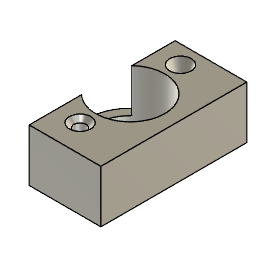
obudowa (Autodesk Fusion 360 archive; units mm, degrees)
design "trzyma_silnik"
Autodesk Fusion 360 part; units mm, degrees
sketch "Sketch1" plane through (0, 0, 0) normal (0, 0, 1) x (1, 0, 0)
  line L0 (22.8277, 15) -> (38.55, 15)
  line L1 (38.55, 15) -> (38.55, -17)
  line L2 (22.8277, -17) -> (22.8277, 15)
  line L3 (38.55, -17) -> (22.8277, -17)
  circle A0 centre (28, 11) radius 1.35
  circle A1 centre (28, 0) radius 7.55
  arc A2 (22.8277, 8.0281) -> (22.8277, -8.0281) centre (28, 0) ccw
  circle A3 centre (28, -11) radius 1.35
  line L4 (22.8277, -39) -> (22.8277, -7)
  point P0 (22.8277, -5.5)
  point P1 (28, 0)
  point P2 (22.8277, 5.5)
  dimension "d27" = 15.1
  dimension "d29" = 10.55
  dimension "d30" = 17
  dimension "d31" = 2.7
  dimension "d32" = 10.55
  dimension "d33" = 15
  dimension "d36" = 11
  dimension "d42" = 0
  dimension "d43" = -22
  constraint coincident P1 A1.centre
  constraint horizontal L0
  constraint vertical L1
  constraint horizontal L3
  constraint vertical L2
  constraint coincident P2 A1
  constraint coincident P2 L2
  constraint coincident P0 A1
  constraint coincident P0 L2
  constraint concentric A1 A2
  constraint coincident L2 A2.end
  constraint coincident L2 A2.start
  measures "d27" diameter of A1
  measures "d29" distance of P1 L1
  measures "d30" distance of P1 L3
  measures "d31" diameter of A0
  measures "d32" distance of A0.centre L1
  measures "d33" distance of P1 L0
  measures "d36" distance of P0 P2
extrude "Extrude1" add sketch "Sketch1" along normal blind 11.5 contours L0 L1 L2 L3 A1 L4
chamfer "Chamfer1" [no effect]
chamfer "Chamfer2" distance 1 distance2 3 1 edges at (26.7414, 11.4882, 11.5) measured on face at (29.8927, -15.4387, 11.5)
chamfer "Chamfer2" distance 1 distance2 1 1 edges at (26.7414, -10.5118, 11.5) measured on face at (29.8927, -15.4387, 11.5)
extrude "Extrude2" add sketch "Sketch1" along normal blind 2 contours L2 A1 A2 L4
equation "d29 = ( 15.1 / 2 ) * 1 mm + 3 mm"

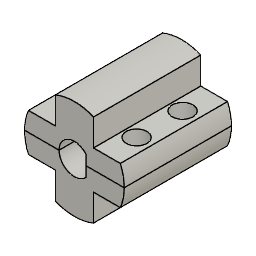
design "laczenie_DC-pret"
part number: laczenie_DC-pret
Autodesk Fusion 360 part; units mm, degrees
sketch "Sketch5" plane through (0, 0, 0) normal (0, 1, 0) x (1, 0, 0)
  circle A0 centre (20, 0) radius 6.5
  circle A1 centre (20, 0) radius 1.45
  line L0 (0, 0) -> (20, 0) construction
  line L1 (20.8832, -1.15) -> (20.8832, 1.15)
  circle A2 centre (20, 0) radius 2
  line L2 (21.5199, -1.3) -> (21.5199, 1.3)
  dimension "d32" = 13
  dimension "d33" = 2.9
  dimension "d34" = 20
  dimension "d37" = 4
  dimension "d39" = 2.6
  dimension "d42" = 2.3
  constraint concentric A0 A1
  constraint coincident L0.start origin
  constraint coincident A0.centre A1.centre
  constraint horizontal L0
  constraint coincident A1 L1.start
  constraint coincident A1 L1.end
  constraint vertical L1
  constraint concentric A1 A2
  constraint coincident A2 L2.start
  constraint coincident A2 L2.end
  constraint parallel L1 L2
  measures "d32" diameter of A0
  measures "d33" diameter of A1
  measures "d34" distance of L0.start A0.centre
  measures "d37" diameter of A2
  measures "d39" distance of L2.start L2.end
  measures "d42" distance of L1.start L1.end
extrude "Extrude9" add sketch "Sketch5" along normal blind 14 contours A0 | A1 L1 | A2 L2 | A2 L2 picked at (21.2814, 0.0105) makes body 1
extrude "Extrude10" cut sketch "Sketch5" along normal blind 7 contours A1 L1 | A2 L2 picked at (21.2814, 0.0105) picked at (18.187, 0) bodies 1
sketch "Sketch6" plane through (0, 0, 0) normal (0, -1, 0) x (1, 0, 0)
  arc A0 (21.5199, 1.3) -> (21.5199, -1.3) centre (20, 0) ccw
  line L0 (21.5199, 1.3) -> (21.5199, -1.3)
  circle A1 centre (20, 0) radius 6.5
  circle A2 centre (20, 0) radius 6.5
  line L1 (17.5, 6) -> (17.5, 2.5)
  line L2 (17.5, 2.5) -> (14, 2.5)
  line L3 (22.5, 6) -> (22.5, 2.5)
  line L4 (22.5, 2.5) -> (26, 2.5)
  line L5 (22.5, -6) -> (22.5, -2.5)
  line L6 (22.5, -2.5) -> (26, -2.5)
  line L7 (17.5, -6) -> (17.5, -2.5)
  line L8 (17.5, -2.5) -> (14, -2.5)
  line L9 (14, 2.5) -> (26, 2.5) construction
  line L10 (14, -2.5) -> (26, -2.5) construction
  line L11 (17.5, 6) -> (17.5, -6) construction
  line L12 (22.5, -6) -> (22.5, 6) construction
  dimension "d45" = 13
  dimension "d46" = 3.5
  constraint concentric A0 A2
  constraint coincident A2 L1.start
  constraint vertical L1
  constraint coincident A1 L2.end
  constraint perpendicular L1 L2
  constraint coincident A2 L3.start
  constraint perpendicular L2 L3
  constraint coincident A1 L4.end
  constraint perpendicular L3 L4
  constraint coincident A2 L5.start
  constraint vertical L5
  constraint coincident A2 L6.end
  constraint perpendicular L5 L6
  constraint coincident A2 L7.start
  constraint perpendicular L6 L7
  constraint coincident A1 L8.end
  constraint perpendicular L7 L8
  constraint perpendicular L3 L9
  constraint parallel L6 L10
  constraint perpendicular L9 L12
  constraint collinear L3 L12
  constraint vertical L11
  constraint equal L9 L12
  constraint equal L9 L11
  constraint equal L10 L11
  measures "d45" diameter of A2
  measures "d46" distance of L1.end L2.end
extrude "Extrude11" cut sketch "Sketch6" against normal blind 22 contours A1 A2 L3 L4 | A1 A2 L5 L6 | A1 A2 L1 L2 | A1 A2 L7 L8 bodies 1
sketch "Sketch7" plane through (0, 0, 2.5) normal (0, 0, 1) x (-1, 0, 0)
  line L0 (-17.5, -14) -> (-14, -14)
  line L1 (-14, -14) -> (-14, 0)
  line L2 (-14, 0) -> (-17.5, 0)
  line L3 (-17.5, 0) -> (-17.5, -14)
  circle A0 centre (-15.925, -10) radius 1.35
  circle A1 centre (-24.12, -10) radius 1.35
  line L4 (-24.12, -10) -> (-24.12, -14) construction
  line L5 (-24.12, -10) -> (-25.82, -10) construction
  line L6 (-15.925, -10) -> (-14.225, -10) construction
  line L7 (-15.925, -10) -> (-15.925, -14) construction
  line L8 (-14, -7) -> (-26, -7) construction
  line L9 (-14, -7) -> (-26, -7) construction
  circle A2 centre (-15.925, -4) radius 1.35
  circle A3 centre (-24.12, -4) radius 1.35
  dimension "d49" = 2.7
  dimension "d50" = 2.7
  dimension "d52" = 4
  dimension "d53" = 1.7
  constraint coincident A1.centre L4.start
  constraint vertical L4
  constraint perpendicular L4 L5
  constraint coincident A0.centre L6.start
  constraint perpendicular L1 L6
  constraint coincident L0 L7.end
  constraint perpendicular L0 L7
  constraint equal L4 L7
  constraint equal L5 L6
  constraint collinear L5 L6
  constraint midpoint L1 L8.start
  constraint perpendicular L1 L8
  constraint symmetric A0 L8 A2
  constraint symmetric A1 L8 A3
  constraint symmetric L9.start L8 L8.start
  constraint symmetric L9.end L8 L8.end
  measures "d49" diameter of A0
  measures "d50" diameter of A1
  measures "d52" distance of A0.centre L7.end
  measures "d53" distance of A0.centre L6.end
extrude "Extrude12" cut sketch "Sketch7" against normal blind 7 contours A0 | A1 | A2 | A3 bodies 1
copy_body "Body->Comp1" bodies 1 removing the originals makes body 2 in component "MaterialInv_072"
ref_plane "WorkPlane1" through (24.25, 7, 0) normal (0, 0, 1) x (1, 0, 0) in component "MaterialInv_072"
split "Split1" by plane through (24.25, 7, 0) normal (0, 0, 1) bodies 2 makes body 3 at (21.4142, 9.3333, 6.3443) in component "MaterialInv_072"
component "MaterialInv_072" placed x (1, 0, 0) y (0, 1, 0) z (0, 0, 1) at (0, 0, 0)
component "MaterialInv_072" placed x (1, 0, 0) y (0, 1, 0) z (0, 0, 1) at (0, 0, 0)
